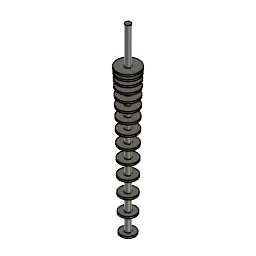
OctoLimb (Autodesk Fusion 360 design; units mm, degrees)
part number: 2026-05-05-22-21-23-308
Autodesk Fusion 360 part; units mm, degrees
sketch "Sketch1" plane through (0, 0, 0) normal (0, 0, 1) x (1, 0, 0)
  circle A0 centre (0, 0) radius 5
extrude "Extrude1" add sketch "Sketch1" along normal blind 330.2 makes body 1
ref_plane "WorkPlane1" through (0, 0, 0) normal (0, 0, 1) x (1, 0, 0)
sketch "Sketch2" plane through (0, 0, 0) normal (0, 0, 1) x (1, 0, 0)
  circle A0 centre (0, 0) radius 13
  circle A1 centre (0, 0) radius 5.1
extrude "Extrude2" add sketch "Sketch2" along normal blind 3 separate body makes body 2
ref_plane "WorkPlane2" through (0, 0, 32) normal (0, 0, 1) x (1, 0, 0)
sketch "Sketch3" plane through (0, 0, 32) normal (0, 0, 1) x (1, 0, 0)
  circle A0 centre (0, 0) radius 14
  circle A1 centre (0, 0) radius 5.1
extrude "Extrude3" add sketch "Sketch3" along normal blind 3 separate body makes body 3
ref_plane "WorkPlane3" through (0, 0, 62) normal (0, 0, 1) x (1, 0, 0)
sketch "Sketch4" plane through (0, 0, 62) normal (0, 0, 1) x (1, 0, 0)
  circle A0 centre (0, 0) radius 14.5
  circle A1 centre (0, 0) radius 5.1
extrude "Extrude4" add sketch "Sketch4" along normal blind 3 separate body makes body 4
ref_plane "WorkPlane4" through (0, 0, 90) normal (0, 0, 1) x (1, 0, 0)
sketch "Sketch5" plane through (0, 0, 90) normal (0, 0, 1) x (1, 0, 0)
  circle A0 centre (0, 0) radius 15
  circle A1 centre (0, 0) radius 5.1
extrude "Extrude5" add sketch "Sketch5" along normal blind 3 separate body makes body 5
ref_plane "WorkPlane5" through (0, 0, 116) normal (0, 0, 1) x (1, 0, 0)
sketch "Sketch6" plane through (0, 0, 116) normal (0, 0, 1) x (1, 0, 0)
  circle A0 centre (0, 0) radius 15.5
  circle A1 centre (0, 0) radius 5.1
extrude "Extrude6" add sketch "Sketch6" along normal blind 3 separate body makes body 6
ref_plane "WorkPlane6" through (0, 0, 140) normal (0, 0, 1) x (1, 0, 0)
sketch "Sketch7" plane through (0, 0, 140) normal (0, 0, 1) x (1, 0, 0)
  circle A0 centre (0, 0) radius 16
  circle A1 centre (0, 0) radius 5.1
extrude "Extrude7" add sketch "Sketch7" along normal blind 3 separate body makes body 7
ref_plane "WorkPlane7" through (0, 0, 162) normal (0, 0, 1) x (1, 0, 0)
sketch "Sketch8" plane through (0, 0, 162) normal (0, 0, 1) x (1, 0, 0)
  circle A0 centre (0, 0) radius 16.5
  circle A1 centre (0, 0) radius 5.1
extrude "Extrude8" add sketch "Sketch8" along normal blind 3 separate body makes body 8
ref_plane "WorkPlane8" through (0, 0, 182) normal (0, 0, 1) x (1, 0, 0)
sketch "Sketch9" plane through (0, 0, 182) normal (0, 0, 1) x (1, 0, 0)
  circle A0 centre (0, 0) radius 17
  circle A1 centre (0, 0) radius 5.1
extrude "Extrude9" add sketch "Sketch9" along normal blind 3 separate body makes body 9
ref_plane "WorkPlane9" through (0, 0, 200) normal (0, 0, 1) x (1, 0, 0)
sketch "Sketch10" plane through (0, 0, 200) normal (0, 0, 1) x (1, 0, 0)
  circle A0 centre (0, 0) radius 17.5
  circle A1 centre (0, 0) radius 5.1
extrude "Extrude10" add sketch "Sketch10" along normal blind 3 separate body makes body 10
ref_plane "WorkPlane10" through (0, 0, 216) normal (0, 0, 1) x (1, 0, 0)
sketch "Sketch11" plane through (0, 0, 216) normal (0, 0, 1) x (1, 0, 0)
  circle A0 centre (0, 0) radius 18
  circle A1 centre (0, 0) radius 5.1
extrude "Extrude11" add sketch "Sketch11" along normal blind 3 separate body makes body 11
ref_plane "WorkPlane11" through (0, 0, 230) normal (0, 0, 1) x (1, 0, 0)
sketch "Sketch12" plane through (0, 0, 230) normal (0, 0, 1) x (1, 0, 0)
  circle A0 centre (0, 0) radius 18.5
  circle A1 centre (0, 0) radius 5.1
extrude "Extrude12" add sketch "Sketch12" along normal blind 3 separate body makes body 12
ref_plane "WorkPlane12" through (0, 0, 242) normal (0, 0, 1) x (1, 0, 0)
sketch "Sketch13" plane through (0, 0, 242) normal (0, 0, 1) x (1, 0, 0)
  circle A0 centre (0, 0) radius 19
  circle A1 centre (0, 0) radius 5.1
extrude "Extrude13" add sketch "Sketch13" along normal blind 3 separate body makes body 13
ref_plane "WorkPlane13" through (0, 0, 252) normal (0, 0, 1) x (1, 0, 0)
sketch "Sketch14" plane through (0, 0, 252) normal (0, 0, 1) x (1, 0, 0)
  circle A0 centre (0, 0) radius 19.5
  circle A1 centre (0, 0) radius 5.1
extrude "Extrude14" add sketch "Sketch14" along normal blind 3 separate body makes body 14
ref_plane "WorkPlane14" through (0, 0, 260) normal (0, 0, 1) x (1, 0, 0)
sketch "Sketch15" plane through (0, 0, 260) normal (0, 0, 1) x (1, 0, 0)
  circle A0 centre (0, 0) radius 20
  circle A1 centre (0, 0) radius 5.1
extrude "Extrude15" add sketch "Sketch15" along normal blind 3 separate body makes body 15
sketch "Sketch16" plane through (0, 0, 0) normal (0, 0, 1) x (1, 0, 0)
  circle A0 centre (6, 0) radius 0.5
extrude "Extrude16" add sketch "Sketch16" along normal blind 330.2 separate body makes body 16
